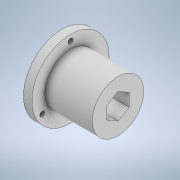
# Autodesk Inventor part: wheel_gearing_mount_long
Saved by Autodesk Inventor 2021 (Build 250183000, 183)
## iProperties
Created: 2021-01-10
Part Number: wheel_gearing_mount_long
Material: Generic
Document SubType Name: Modeling
Designer: Mateusz
Density: 1 g/cm^3
Appearance: Default
Author: Mateusz
Autodesk Inventor part; units mm, degrees
ref_plane "YZ Plane" through (0, 0, 0) normal (1, 0, 0) x (0, 1, 0)
ref_plane "XZ Plane" through (0, 0, 0) normal (0, 1, 0) x (-1, 0, 0)
ref_plane "XY Plane" through (0, 0, 0) normal (0, 0, 1) x (1, 0, 0)
sketch "Sketch1" plane through (0, 0, 0) normal (1, 0, 0) x (0, 1, 0)
  circle A0 centre (0, 0) radius 15
  line L0 (0, 0) -> (7.5, 0)
  line L1 (7.5, 0) -> (3.75, -6.4952)
  line L2 (3.75, -6.4952) -> (-3.75, -6.4952)
  line L3 (-3.75, -6.4952) -> (-7.5, 0)
  line L4 (-7.5, 0) -> (-3.75, 6.4952)
  line L5 (-3.75, 6.4952) -> (3.75, 6.4952)
  line L6 (3.75, 6.4952) -> (7.5, 0)
  dimension "d0" = 30
  dimension "d1" = 7.5
  constraints: 14 end point, 2 coincident, 1 centre point, 1 horizontal, 13 other
  measures "d0" diameter of A0
  measures "d1" distance of L0.start L0.end
extrude "Extrusion1" add sketch "Sketch1" along normal blind 32.75
sketch "Sketch2" plane through (0, 0, 0) normal (-1, 0, 0) x (0, 0, 1)
  circle A0 centre (0, 0) radius 22.5
  line L0 (0, 7.5) -> (-6.4952, 3.75) projected
  line L1 (-6.4952, 3.75) -> (-6.4952, -3.75) projected
  line L2 (-6.4952, -3.75) -> (0, -7.5) projected
  line L3 (0, -7.5) -> (6.4952, -3.75) projected
  line L4 (6.4952, -3.75) -> (6.4952, 3.75) projected
  line L5 (6.4952, 3.75) -> (0, 7.5) projected
  dimension "d4" = 45
  constraints: 1 centre point, 1 coincident
  measures "d4" diameter of A0
extrude "Extrusion2" add sketch "Sketch2" against normal blind 5
sketch "Sketch3" plane through (0, 0, 0) normal (-1, 0, 0) x (0, 0, 1)
  circle A0 centre (0, 19.05) radius 1.45
  circle A1 centre (-16.4978, -9.525) radius 1.45
  circle A2 centre (16.4978, -9.525) radius 1.45
  point P0 (0, 0)
  dimension "d11" = 360
  constraints: 3 centre point, 7 other
extrude "Extrusion3" cut sketch "Sketch3" against normal up to surface (5 mm away)
sketch "Sketch4" plane through (0, 0, 0) normal (-1, 0, 0) x (0, 0, 1)
  line L0 (6.4952, 3.75) -> (0, 7.5) projected
  circle A0 centre (0, 0) radius 7.5
  constraints: 1 coincident, 1 vertical alignment, 2 other
body "Solid1"
